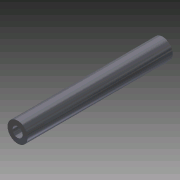
# Autodesk Inventor part: Roller Axle V4 1764
Saved by Autodesk Inventor 2011 (Build 150239000, 239)
## iProperties
Created: 2007-11-28
Part Number: Roller Axle V4 1764
Document SubType Name: Modeling
Designer: lwoods
Density: 7.84 g/cm^3
Material: Steel, High Strength Low Alloy
Mass: 10.4976 g
Surface Area: 11.0198 cm^2
Volume: 1.33898 cm^3
Author: lwoods
Autodesk Inventor part; units mm, degrees
ref_plane "YZ Plane" through (0, 0, 0) normal (1, 0, 0) x (0, 1, 0)
ref_plane "XZ Plane" through (0, 0, 0) normal (0, 1, 0) x (-1, 0, 0)
ref_plane "XY Plane" through (0, 0, 0) normal (0, 0, 1) x (1, 0, 0)
sketch "Sketch1" plane through (0, 0, 0) normal (0, 0, 1) x (1, 0, 0)
  circle A0 centre (-19.5853, 0.9985) radius 3.1623
  dimension "d0" = 6.3246
  constraints: 1 centre point
  measures "d0" diameter of A0
extrude "Extrusion1" add sketch "Sketch1" against normal blind 45.8724
sketch "Sketch2" plane through (-19.5853, 0.9985, 0) normal (0, 0, 1) x (1, 0, 0)
  circle A0 centre (0, 0) radius 3.1623 projected
  circle A1 centre (0, 0) radius 1.6002
  dimension "d3" = 3.2004
  constraints: 1 centre point, 1 coincident
  measures "d3" diameter of A1
extrude "Extrusion2" cut sketch "Sketch2" against normal blind 6.35 contours A1
sketch "Sketch3" plane through (-19.5853, 0.9985, -45.8724) normal (0, 0, -1) x (-1, 0, 0)
  circle A0 centre (0, 0) radius 3.1623 projected
  circle A1 centre (0, 0) radius 1.6002
  dimension "d6" = 3.2004
  constraints: 1 centre point, 1 coincident
  measures "d6" diameter of A1
extrude "Extrusion3" cut sketch "Sketch3" against normal blind 6.35 contours A1
body "Solid1"
